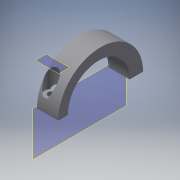
# Autodesk Inventor part: 04_Tubeholder_top
Saved by Autodesk Inventor 2016 (Build 200138000, 138)
## iProperties
Created: 2016-09-10
Part Number: 04_Tubeholder_top
Material: Generisch
Document SubType Name: Modeling
Designer: Bene
Density: 1 g/cm^3
Appearance: Vorgabe
Mass: 2.47764 g
Surface Area: 19.404 cm^2
Volume: 2.47764 cm^3
Author: Bene
Autodesk Inventor part; units mm, degrees
ref_plane "YZ Plane" through (0, 0, 0) normal (1, 0, 0) x (0, 1, 0)
ref_plane "XZ Plane" through (0, 0, 0) normal (0, 1, 0) x (-1, 0, 0)
ref_plane "XY Plane" through (0, 0, 0) normal (0, 0, 1) x (1, 0, 0)
ref_plane "Arbeitsebene1" through (-5, 20, -19) normal (-1, 0, 0) x (0, -1, 0)
sketch "Skizze1" plane through (-5, 20, -19) normal (-1, 0, 0) x (0, -1, 0)
  arc A0 (6.3684, 19) -> (35.3565, 19) centre (20.8625, 19.5) ccw projected
  line L0 (0, 19) -> (6.3684, 19) projected
  line L1 (0, 0) -> (0, 19) projected
  line L2 (0, 0) -> (40, 0) projected
  line L3 (40, 0) -> (40, 19) projected
  line L4 (35.3565, 19) -> (40, 19) projected
  circle A1 centre (20.8625, 19.5) radius 14.5027
  arc A2 (40, 19) -> (0, 19) centre (20, 19) ccw
  point P0 (20, 19)
  constraints: 2 centre point, 2 point on circle, 2 tangent, 1 coincident, 1 concentric
ref_plane "Arbeitsebene2" through (5, -20, -19) normal (1, 0, 0) x (0, 1, 0)
extrude "Extrusion1" add sketch "Skizze1" against normal up to surface (10 mm away) contours L0 A2 L4 A1
sketch "Skizze2" plane through (-5, 13.6316, 0) normal (0, 0, -1) x (-1, 0, 0)
  circle A0 centre (-3, 3.5086) radius 1.5 projected
  circle A1 centre (-3, -29.9914) radius 1.5 projected
  point P0 (-5, -13.6316)
extrude "Extrusion2" cut sketch "Skizze2" against normal through all
ref_plane "Arbeitsebene3" through (-5, -20, 19.5) normal (0, 0, -1) x (-1, 0, 0)
sketch "Skizze3" plane through (-5, -20, 19.5) normal (0, 0, -1) x (-1, 0, 0)
  spline S0 degree 5 poles (-1.5, 37.1402) (-1.5, 37.2612) (-1.5119, 37.3788) (-1.535, 37.4929) (-1.5686, 37.6029) (-1.6903, 37.9001) (-1.797, 38.0668) (-1.931, 38.2268) (-2.1133, 38.3781) (-2.4019, 38.5171) (-2.4579, 38.5408) (-2.5176, 38.5628) (-2.5815, 38.5824) (-2.7136, 38.6141) (-2.7811, 38.6267) (-2.8524, 38.6356) (-2.9262, 38.6402) (-3.0947, 38.6402) (-3.1873, 38.6328) (-3.2762, 38.6184) (-3.3593, 38.5987) (-3.5324, 38.5463) (-3.6204, 38.5105) (-3.6998, 38.471) (-3.7719, 38.4289) (-4.0013, 38.2742) (-4.133, 38.1466) (-4.2378, 38.0111) (-4.3223, 37.868) (-4.4551, 37.5466) (-4.4988, 37.3703) (-4.5173, 37.1838) (-4.5063, 36.9891) (-4.422, 36.6378) (-4.3641, 36.4834) (-4.2806, 36.3279) (-4.1672, 36.1769) (-3.9148, 35.9428) (-3.7929, 35.8527) (-3.6522, 35.7746) (-3.495, 35.7139) (-3.1755, 35.6424) (-3.015, 35.6273) (-2.853, 35.6345) (-2.6962, 35.6634) (-2.4232, 35.7491) (-2.3041, 35.8022) (-2.1956, 35.8653) (-2.0985, 35.9359) (-1.7804, 36.2143) (-1.6274, 36.4535) (-1.5406, 36.69) (-1.5, 36.9204) (-1.5, 37.1402) knots 0 0 0 0 0 0 0.074792 0.074792 0.074792 0.074792 0.210061 0.210061 0.210061 0.210061 0.240207 0.240207 0.240207 0.240207 0.268288 0.268288 0.268288 0.268288 0.30433 0.30433 0.30433 0.30433 0.351064 0.351064 0.351064 0.351064 0.465013 0.465013 0.465013 0.465013 0.586915 0.586915 0.586915 0.586915 0.680147 0.680147 0.680147 0.680147 0.746463 0.746463 0.746463 0.746463 0.806674 0.806674 0.806674 0.806674 0.859155 0.859155 0.859155 0.859155 1 1 1 1 1 1 projected
  spline S1 degree 5 poles (-1.5, 3.6402) (-1.5, 3.848) (-1.5358, 4.0635) (-1.6138, 4.284) (-1.7415, 4.4986) (-2.0339, 4.7977) (-2.1588, 4.8982) (-2.3031, 4.9848) (-2.464, 5.0522) (-2.7782, 5.1311) (-2.9287, 5.1501) (-3.0815, 5.1495) (-3.2318, 5.1295) (-3.6761, 5.0149) (-3.9459, 4.8609) (-4.1443, 4.66) (-4.2864, 4.4472) (-4.4768, 4.0017) (-4.5201, 3.7705) (-4.5202, 3.5456) (-4.4835, 3.3326) (-4.3603, 2.9904) (-4.292, 2.8562) (-4.2061, 2.7283) (-4.1012, 2.6082) (-3.9053, 2.4408) (-3.8296, 2.3851) (-3.7463, 2.3332) (-3.6543, 2.286) (-3.4933, 2.2222) (-3.4301, 2.2009) (-3.3638, 2.1825) (-3.2944, 2.1676) (-3.1123, 2.1403) (-2.9961, 2.1334) (-2.8796, 2.1383) (-2.7674, 2.1545) (-2.5579, 2.2028) (-2.4605, 2.2352) (-2.371, 2.2736) (-2.2891, 2.3164) (-2.0153, 2.485) (-1.8583, 2.6347) (-1.738, 2.7959) (-1.6452, 2.9671) (-1.5495, 3.2456) (-1.5251, 3.3409) (-1.5085, 3.4386) (-1.5, 3.5385) (-1.5, 3.6402) knots 0 0 0 0 0 0 0.129492 0.129492 0.129492 0.129492 0.203677 0.203677 0.203677 0.203677 0.265882 0.265882 0.265882 0.265882 0.397044 0.397044 0.397044 0.397044 0.534696 0.534696 0.534696 0.534696 0.63201 0.63201 0.63201 0.63201 0.685078 0.685078 0.685078 0.685078 0.716299 0.716299 0.716299 0.716299 0.764042 0.764042 0.764042 0.764042 0.811806 0.811806 0.811806 0.811806 0.937436 0.937436 0.937436 0.937436 1 1 1 1 1 1 projected
  line L0 (-10, 0) -> (-10, 40) projected
  line L1 (0, 40) -> (-10, 40) projected
  line L2 (0, 0) -> (0, 40) projected
  line L3 (0, 0) -> (-10, 0) projected
  spline S2 degree 5 poles (0, 3.6402) (-0.0008, 4.6577) (-0.4287, 5.6783) (-1.3024, 6.4454) (-3.3765, 7.0278) (-5.2462, 5.9892) (-5.8957, 5.1159) (-6.329, 3.1357) (-5.3147, 1.3987) (-4.5017, 0.7892) (-2.648, 0.328) (-0.9517, 1.1808) (-0.3152, 1.8974) (-0.0002, 2.769) (0, 3.6402) knots 0 0 0 0 0 0 0.270032 0.270032 0.270032 0.526397 0.526397 0.526397 0.768893 0.768893 0.768893 1 1 1 1 1 1
  spline S3 degree 5 poles (0, 37.1402) (0.0001, 37.9886) (-0.2992, 38.8371) (-0.9019, 39.543) (-2.5377, 40.4271) (-4.373, 40.0502) (-5.2031, 39.4853) (-6.2923, 37.8166) (-5.9721, 35.8338) (-5.3794, 34.9312) (-3.55, 33.763) (-1.4028, 34.2504) (-0.4611, 35.0252) (-0.0009, 36.0847) (0, 37.1402) knots 0 0 0 0 0 0 0.225035 0.225035 0.225035 0.465161 0.465161 0.465161 0.719843 0.719843 0.719843 1 1 1 1 1 1
  point P0 (-5, 20)
  dimension "d5" = 1.5
  dimension "d6" = 1.5
  constraints: 6 other
extrude "Extrusion3" cut sketch "Skizze3" along normal blind 14 contours S0 | S1 | S2 | S3 L1 | L1 S3
